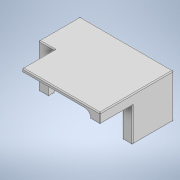
# Autodesk Inventor part: OBS-SnapInPCBHolder
Saved by Autodesk Inventor 2020.3 (Build 243373000, 373)
## iProperties
Created: 2020-06-21
Part Number: OBS-SnapInPCBHolder
Material: Generisch
Document SubType Name: Modeling
Designer: hpcwoess
Density: 1 g/cm^3
Appearance: Vorgabe
Author: hpcwoess
Autodesk Inventor part; units mm, degrees
ref_plane "YZ Plane" through (0, 0, 0) normal (1, 0, 0) x (0, 1, 0)
ref_plane "XZ Plane" through (0, 0, 0) normal (0, 1, 0) x (-1, 0, 0)
ref_plane "XY Plane" through (0, 0, 0) normal (0, 0, 1) x (1, 0, 0)
sketch "Skizze1" plane through (0, 0, 0) normal (0, 0, 1) x (1, 0, 0)
  line L0 (-24.8, -23.2) -> (-24.8, 0)
  line L1 (-24.8, 0) -> (24.8, 0)
  line L2 (24.8, 0) -> (24.8, -23.2)
  line L3 (24.8, -23.2) -> (19.5, -23.2)
  line L4 (19.5, -23.2) -> (19.5, -2)
  line L5 (19.5, -2) -> (-19.5, -2)
  line L6 (-19.5, -2) -> (-19.5, -23.2)
  line L7 (-19.5, -23.2) -> (-24.8, -23.2)
  point P0 (0, 0)
  dimension "d0" = 49.6
  dimension "d1" = 23.2
  dimension "d2" = 2
  dimension "d3" = 39
  dimension "d4" = 5.3
  dimension "d5" = 5.3
  dimension "d6" = 24.8
  constraints: 16 end point, 7 perpendicular, 1 midpoint, 1 point on line, 1 vertical
  measures "d0" distance of L0.end L1.end
  measures "d1" distance of L1.end L2.end
  measures "d2" distance between parallel lines of L1 L5
  measures "d3" distance between parallel lines of L4 L6
  measures "d4" distance between parallel lines of L2 L4
  measures "d5" distance of L6.end L0.start
  measures "d6" distance from line of L2 point (0, 0)
extrude "Extrusion1" add sketch "Skizze1" along normal blind 22
sketch "Skizze2" plane through (0, 0, 0) normal (0, 0, -1) x (-1, 0, 0)
  line L0 (24.8, -23.2) -> (19.5, -23.2) projected
  line L1 (21.7, -23.2) -> (-21.7, -23.2)
  line L2 (-21.7, -23.2) -> (-21.7, -2)
  line L3 (-21.7, -2) -> (21.7, -2)
  line L4 (21.7, -2) -> (21.7, -23.2)
  line L5 (19.5, -2) -> (-19.5, -2) projected
  point P0 (0, 0)
  dimension "d9" = 43.4
  dimension "d10" = 21.7
  constraints: 8 end point, 2 collinear, 2 parallel, 1 horizontal, 1 perpendicular
  measures "d9" distance between parallel lines of L2 L4
  measures "d10" distance from line of L4 point (0, 0)
extrude "Extrusion2" cut sketch "Skizze2" against normal blind 14.5
fillet "Rundung1" radius 3 4 edges at (-21.7, -2, 7.25) (-19.5, -2, 18.25) (19.5, -2, 18.25) (21.7, -2, 7.25)
sketch "Skizze3" plane through (19.5, -23.2, 22) normal (0, -1, 0) x (1, 0, 0)
  line L0 (-40.5, -3) -> (1.5, -3)
  line L1 (1.5, -3) -> (1.5, -5)
  line L2 (1.5, -5) -> (-40.5, -5)
  line L3 (-40.5, -5) -> (-40.5, -3)
  line L4 (-42.5, -10) -> (3.5, -10)
  line L5 (3.5, -10) -> (3.5, -12)
  line L6 (3.5, -12) -> (-42.5, -12)
  line L7 (-42.5, -12) -> (-42.5, -10)
  line L8 (-0.8, -22) -> (-38.2, -22) projected
  line L9 (0, -7.5) -> (2.2, -7.5) projected
  point P0 (-19.5, -22)
  dimension "d14" = 10
  dimension "d15" = 2
  dimension "d16" = 2
  dimension "d17" = 2.5
  dimension "d18" = 42
  dimension "d19" = 21
  dimension "d20" = 46
  dimension "d21" = 23
  constraints: 16 end point, 4 parallel, 2 horizontal, 2 perpendicular
  measures "d14" distance between parallel lines of L8 L6
  measures "d15" distance between parallel lines of L6 L4
  measures "d16" distance between parallel lines of L0 L2
  measures "d17" distance between parallel lines of L2 L9
  measures "d18" distance of L0.start L0.end
  measures "d19" distance from line of point (-19.5, -22) L1
  measures "d20" distance of L5.end L6.end
  measures "d21" distance from line of point (-19.5, -22) L7
extrude "Extrusion3" cut sketch "Skizze3" against normal up to surface (21.2 mm away)
sketch "Skizze4" plane through (0, 0, 22) normal (0, 0, 1) x (1, 0, 0)
  line L0 (24.8, 0) -> (-24.8, 0) projected
  line L1 (19.5, -5) -> (19.5, -23.2) projected
  line L2 (24.8, 0) -> (19.5, 0)
  line L3 (19.5, 0) -> (19.5, -5.3)
  line L4 (19.5, -5.3) -> (24.8, -5.3)
  line L5 (24.8, -5.3) -> (24.8, 0)
  arc A0 (-16.5, -2) -> (-19.5, -5) centre (-16.5, -5) ccw projected
  line L6 (19.5, 0) -> (-16.5, 0)
  line L7 (-16.5, 0) -> (-16.5, -2)
  line L8 (-16.5, -2) -> (19.5, -2)
  line L9 (19.5, -2) -> (19.5, 0)
  point P0 (0, 0)
  dimension "d24" = 5.3
  constraints: 16 end point, 4 parallel, 2 horizontal, 2 perpendicular, 1 point on line
  measures "d24" distance of L4.end L0.start
extrude "Extrusion4" add sketch "Skizze4" along normal blind 17
fillet "Rundung2" radius 3 1 edges at (19.5, -2, 30.5)
fillet "Rundung3" radius 0.5 21 edges at (-24.8, -11.6, 22) (-22.15, -23.2, 22) (-23.25, -23.2, 0) (-24.8, -11.6, 0) (-23, -23.2, 11) (-22.35, -23.2, 12) (-22.35, -23.2, 10) (-20.6, -23.2, 14.5) (-21.7, -23.2, 13.25) (-21.7, -23.2, 5) (-19.5, -23.2, 15.75) (-20.25, -23.2, 17) (-21, -23.2, 18) (-20.25, -23.2, 19) (-19.5, -23.2, 20.5) (-24.8, -23.2, 11) (19.5, -23.2, 20.5) (20.25, -23.2, 19) (21, -23.2, 18) (20.25, -23.2, 17) (19.5, -23.2, 15.75)
fillet "Rundung4" radius 0.5 38 edges at (19.6464, -23.0536, 14.5) (19.5, -13.85, 14.5) (18.6213, -2.8787, 14.5) (20.85, -23.2, 14.5) (21.7, -23.2, 13.25) (22.35, -23.2, 12) (23, -23.2, 11) (22.35, -23.2, 10) (21.7, -23.2, 5) (19.6464, -23.0536, 22) (19.5, -14, 22) (22.4, -23.2, 22) (24.8, -23.2, 11) (23.25, -23.2, 0) (20.8213, -2.8787, 0) (0, -2, 0) (-20.8213, -2.8787, 0) (-21.7, -13.85, 0) (-21.8464, -23.0536, 0.1464) (21.7, -14.1, 0) (-24.6536, 0, 0.1464) (-24.8, 0, 11) (-24.6536, 0, 21.8536) (-20.4, 0, 22) (0.25, 0, 0) (24.8, -11.6, 0) (24.8, -14.25, 22) (24.8, -5.3, 30.5) (24.8, 0, 19.5) (-16.5, 0, 30.5) (4.15, 0, 39) (24.8, -2.65, 39) (22.15, -5.3, 39) (0, -2, 39) (19.5, -5.15, 39) (18.6213, -2.8787, 39) (-16.5, -1, 39) (-16.5, -2, 30.5)
equation "\"d4\" = d5"
equation "\"d6\" = 0.5 * d0"
equation "\"d10\" = 0.5 * d9"
equation "\"d19\" = 0.5 * d18"
equation "\"d21\" = 0.5 * d20"
